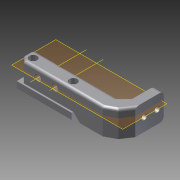
# Autodesk Inventor part: Support Extruder
Saved by Autodesk Inventor 2012 (Build 160160000, 160)
## iProperties
Created: 2013-02-25
Part Number: Support Extruder
Material: Default
Document SubType Name: Modeling
Designer: mce
Density: 1 g/cm^3
Author: mce
Autodesk Inventor part; units mm, degrees
ref_plane "YZ Plane" through (0, 0, 0) normal (1, 0, 0) x (0, 1, 0)
ref_plane "XZ Plane" through (0, 0, 0) normal (0, 1, 0) x (-1, 0, 0)
ref_plane "XY Plane" through (0, 0, 0) normal (0, 0, 1) x (1, 0, 0)
sketch "Sketch1" plane through (0, 0, 0) normal (0, 0, 1) x (1, 0, 0)
  line L0 (3.2057, 1.8441) -> (73.2057, 1.8441)
  line L1 (73.2057, 1.8441) -> (81.2057, 13.8441)
  line L2 (3.2057, 13.8441) -> (3.2057, 1.8441)
  line L3 (73.2057, 18.8441) -> (73.2057, 35.8441)
  line L4 (73.2057, 35.8441) -> (81.2057, 35.8441)
  line L5 (81.2057, 35.8441) -> (81.2057, 13.8441)
  arc A0 (18.1952, 13.8441) -> (30.6162, 13.8441) centre (24.4057, 23.0441) ccw
  line L6 (68.2057, 13.8441) -> (30.6162, 13.8441)
  line L7 (18.1952, 13.8441) -> (3.2057, 13.8441)
  line L8 (73.2057, 18.8441) -> (68.2057, 13.8441)
  circle A1 centre (8.9057, 7.3441) radius 1.6
  circle A2 centre (39.9057, 7.3441) radius 1.6
  point P0 (73.2057, 13.8441)
  dimension "d0" = 70
  dimension "d2" = 8
  dimension "d4" = 21.2
  dimension "d5" = 21.2
  dimension "d6" = 22.2
  dimension "d7" = 12
  dimension "d8" = 22
  dimension "d9" = 5
  dimension "d10" = 5
  dimension "d11" = 31
  dimension "d12" = 5.7
  dimension "d13" = 3.2
  dimension "d14" = 5.5
  constraints: 18 end point, 4 point on line, 3 centre point, 2 point on circle, 1 collinear, 1 equal radius, 1 horizontal, 1 horizontal alignment, 1 vertical, 1 other
  measures "d0" distance between parallel lines of L2 L3
  measures "d2" distance between parallel lines of L3 L5
  measures "d4" distance from line of L0 A0.centre
  measures "d5" distance from line of L2 A0.centre
  measures "d6" diameter of A0
  measures "d7" distance between parallel lines of L7 L0
  measures "d8" distance between parallel lines of L4 L6
  measures "d9" distance of L3.start point (73.206, 13.844)
  measures "d10" distance of L6.start point (73.206, 13.844)
  measures "d11" distance of A1.centre A2.centre
  measures "d12" distance from line of L2 A1.centre
  measures "d13" diameter of A1
  measures "d14" distance from line of A1.centre L0
extrude "Extrusion1" add sketch "Sketch1" along normal blind 20
sketch "Sketch2" plane through (81.2057, 13.8441, 0) normal (1, 0, 0) x (0, 0, -1)
  line L0 (-20, 22) -> (-20, 0) projected
  line L1 (0, 22) -> (-20, 22) projected
  circle A0 centre (-10, 17) radius 2.1
  circle A1 centre (-10, 7) radius 2.1
  point P0 (0, -13.8441)
  dimension "d17" = 10
  dimension "d18" = 4.2
  dimension "d19" = 10
  dimension "d20" = 5
  constraints: 2 centre point, 1 equal radius, 1 vertical alignment
  measures "d17" distance from line of L0 A0.centre
  measures "d18" diameter of A0
  measures "d19" distance of A0.centre A1.centre
  measures "d20" distance from line of L1 A0.centre
extrude "Extrusion2" cut sketch "Sketch2" against normal up to next
sketch "Sketch3" plane through (73.2057, 18.8441, 0) normal (-1, 0, 0) x (0, 0, 1)
  circle A0 centre (10, 2) radius 2.1 projected
  circle A1 centre (10, 12) radius 2.1 projected
  arc A2 (13.75, 12) -> (6.25, 12) centre (10, 12) ccw
  arc A3 (6.25, 2) -> (13.75, 2) centre (10, 2) ccw
  line L0 (6.25, 12) -> (6.25, 2)
  line L1 (13.75, 12) -> (13.75, 2)
  point P0 (0, -18.8441)
  dimension "d23" = 7.5
  constraints: 4 end point, 4 point on circle, 3 tangent, 2 centre point, 2 coincident, 1 equal radius, 1 parallel
  measures "d23" diameter of A2
extrude "Extrusion3" cut sketch "Sketch3" along normal blind 10 and the other way blind 4 contours A0 | L1 A3 L0 A2
sketch "Sketch4" plane through (3.2057, 1.8441, 0) normal (0, -1, 0) x (1, 0, 0)
  line L0 (0, 0) -> (0, 20) projected
  line L1 (0, 0) -> (70, 0) projected
  arc A0 (13.7, 8.5) -> (13.7, 3.5) centre (13.7, 6) ccw
  arc A1 (28.7, 3.5) -> (28.7, 8.5) centre (28.7, 6) ccw
  line L2 (13.7, 8.5) -> (28.7, 8.5)
  line L3 (13.7, 3.5) -> (28.7, 3.5)
  point P0 (-3.2057, 0)
  dimension "d28" = 5
  dimension "d29" = 6
  dimension "d30" = 15
  dimension "d31" = 13.7
  constraints: 4 end point, 4 point on circle, 2 centre point, 2 horizontal, 1 equal radius, 1 horizontal alignment
  measures "d28" diameter of A0
  measures "d29" distance from line of L1 A0.centre
  measures "d30" distance of A1.centre A0.centre
  measures "d31" distance from line of L0 A0.centre
extrude "Extrusion4" [suppressed]
sketch "Sketch5" plane through (3.2057, 1.8441, 0) normal (0, -1, 0) x (1, 0, 0)
  line L0 (0, 0) -> (0, 20) projected
  line L1 (0, 0) -> (70, 0) projected
  circle A0 centre (14.7, 14) radius 1
  circle A1 centre (27.7, 14) radius 1
  point P0 (-3.2057, 0)
  dimension "d34" = 13
  dimension "d35" = 14.7
  dimension "d36" = 14
  dimension "d37" = 2
  constraints: 2 centre point, 1 equal radius, 1 horizontal alignment
  measures "d34" distance of A1.centre A0.centre
  measures "d35" distance from line of L0 A0.centre
  measures "d36" distance from line of L1 A0.centre
  measures "d37" diameter of A0
extrude "Extrusion5" cut sketch "Sketch5" against normal up to next
sketch "Sketch6" plane through (3.2057, 1.8441, 0) normal (0, -1, 0) x (1, 0, 0)
  circle A0 centre (27.7, 14) radius 1 projected
  circle A1 centre (14.7, 14) radius 1 projected
  circle A2 centre (14.7, 14) radius 2.1
  circle A3 centre (27.7, 14) radius 2.1
  point P0 (-3.2057, 0)
  dimension "d40" = 4.2
  constraints: 2 centre point, 2 coincident, 1 equal radius
  measures "d40" diameter of A2
extrude "Extrusion6" cut sketch "Sketch6" against normal blind 4
chamfer "Chamfer1" distance 3 angle 30 2 edges at (31.5017, 13.8441, 13.197) (31.5017, 13.8441, 14.803) measured on face at (31.5017, 13.3441, 14.803) measured on face at (31.5017, 13.3441, 13.197)
chamfer "Chamfer2" distance 3 angle 30 1 edges at (16.9057, 13.8441, 14) measured on face at (16.9057, 13.3441, 14)
chamfer "Chamfer3" distance 5 angle 45 1 edges at (73.2057, 1.8441, 10)
chamfer "Chamfer4" distance 4 angle 45 1 edges at (3.2057, 1.8441, 10)
fillet "Fillet1" radius 3 2 edges at (77.2057, 35.8441, 20) (77.2057, 35.8441, 0)
fillet "Fillet2" radius 3 1 edges at (49.4109, 13.8441, 20)
ref_plane "Work Plane1" through (0, 0, 14) normal (0, 0, 1) x (1, 0, 0)
sketch "Sketch10" plane through (0, 0, 14) normal (0, 0, 1) x (1, 0, 0)
  line L0 (15.8057, 1.8441) -> (15.8057, 1.0941)
  line L1 (15.8057, 1.0941) -> (15.1562, 1.4691)
  line L2 (15.1562, 1.4691) -> (15.8057, 1.8441)
  line L3 (13.7777, 1.4691) -> (17.3129, 1.4691) construction
  line L4 (20.0057, 1.8441) -> (15.8057, 1.8441) projected
  point P0 (0, 0)
  dimension "d80" = 60
  dimension "d81" = 0.75
  dimension "d82" = 0
  constraints: 8 end point, 2 point on line, 1 horizontal, 1 symmetric about line
  measures "d80" angle of L1 L2
  measures "d81" distance of L0.start L0.end
  measures "d82" distance of L0.start L4.end
coil "Coil2" sketch "Sketch10" operation cut axis through (17.9057, 1.8441, 14) along (0, 1, 0) pitch 0.8 turns 5.25 hand right
sketch "Sketch12" plane through (0, 0, 14) normal (0, 0, 1) x (1, 0, 0)
  line L0 (28.8057, 1.8441) -> (28.1562, 1.4691)
  line L1 (28.1562, 1.4691) -> (28.8057, 1.0941)
  line L2 (28.8057, 1.0941) -> (28.8057, 1.8441)
  line L3 (26.005, 1.4691) -> (30.2865, 1.4691) construction
  line L4 (33.0057, 1.8441) -> (28.8057, 1.8441) construction
  point P0 (0, 0)
  dimension "d94" = 60
  dimension "d95" = 0.75
  dimension "d96" = 0
  constraints: 8 end point, 2 point on line, 1 horizontal, 1 symmetric about line
  measures "d94" angle of L0 L1
  measures "d95" distance of L1.end L0.start
  measures "d96" distance of L0.start L4.end
coil "Coil3" sketch "Sketch12" operation cut axis through (30.9057, 1.8441, 14) along (0, 1, 0) pitch 0.8 turns 5.25 hand right
sketch "Sketch13" plane through (0, 0, 20) normal (0, 0, 1) x (1, 0, 0)
  circle A0 centre (39.9057, 7.3441) radius 1.6 projected
  circle A1 centre (8.9057, 7.3441) radius 1.6 projected
  circle A2 centre (8.9057, 7.3441) radius 3
  circle A3 centre (39.9057, 7.3441) radius 3
  point P0 (0, 0)
  dimension "d105" = 6
  constraints: 2 centre point, 2 coincident, 1 equal radius
  measures "d105" diameter of A2
extrude "Extrusion9" cut sketch "Sketch13" against normal blind 4
fillet "Fillet3" radius 2 7 edges at (69.2057, 14.8441, 20) (73.2057, 34.9654, 19.1213) (73.2057, 35.8441, 10) (73.2057, 34.9654, 0.8787) (73.2057, 25.8441, 0) (73.2057, 25.8441, 20) (70.7057, 16.3441, 0)
fillet "Fillet4" radius 2 7 edges at (37.7057, 1.8441, 20) (72.0924, 3.9242, 20) (78.5924, 9.9242, 20) (5.2057, 3.8441, 20) (3.2057, 12.9654, 19.1213) (3.2057, 8.3441, 20) (3.2057, 13.8441, 8.5)
sketch "Sketch14" plane through (0, 0, 0) normal (0, 0, -1) x (-1, 0, 0)
  circle A0 centre (-8.9057, 7.3441) radius 1.6 projected
  circle A1 centre (-39.9057, 7.3441) radius 1.6 projected
  line L0 (-71.0341, 13.8441) -> (-30.6162, 13.8441) projected
  line L1 (-7.2057, 1.8441) -> (-68.2057, 1.8441) projected
  line L2 (-3.2057, 11.8441) -> (-3.2057, 5.8441) projected
  line L3 (-45.6057, 18.8441) -> (1.7943, 18.8441)
  line L4 (1.7943, 18.8441) -> (1.7943, -3.1559)
  line L5 (1.7943, -3.1559) -> (-45.6057, -3.1559)
  line L6 (-45.6057, -3.1559) -> (-45.6057, 18.8441)
  point P0 (0, 0)
  dimension "d110" = 5
  dimension "d111" = 5
  dimension "d112" = 5
  dimension "d113" = 42.4
  constraints: 8 end point
  measures "d110" distance between parallel lines of L3 L0
  measures "d111" distance between parallel lines of L5 L1
  measures "d112" distance between parallel lines of L4 L2
  measures "d113" distance between parallel lines of L6 L2
extrude "Extrusion10" cut sketch "Sketch14" against normal blind 5
chamfer "Chamfer5" distance 5 angle 45 1 edges at (45.6057, 7.8441, 0)
sketch "Sketch16" plane through (30.9057, 13.8441, 14) normal (0, 1, 0) x (1, 0, 0)
  line L0 (14.7, 9) -> (-0.2895, 9) projected
  line L1 (40.1284, 14) -> (19.7, 14) projected
  line L2 (-28.2, 14) -> (14.2, 14)
  line L3 (14.2, 14) -> (14.2, 9.25)
  line L4 (14.2, 9.25) -> (-28.2, 9.25)
  line L5 (-28.2, 9.25) -> (-28.2, 14)
  line L6 (-27.7, 9) -> (-27.7, -3) projected
  point P0 (-30.9057, 14)
  dimension "d119" = 0.5
  dimension "d121" = 0.25
  dimension "d122" = 0.5
  constraints: 8 end point, 1 collinear
  measures "d119" distance from line of L3 L0.start
  measures "d121" distance between parallel lines of L4 L0
  measures "d122" distance between parallel lines of L5 L6
extrude "Extrusion11" add sketch "Sketch16" against normal blind 13 and the other way blind 1
sketch "Sketch17" plane through (45.1057, 0.8441, 0) normal (0, 0, -1) x (-1, 0, 0)
  line L0 (0, 0) -> (42.4, 0) projected
  line L1 (42.4, 0) -> (42.4, 14) projected
  line L2 (42.4, 14) -> (0, 14) projected
  line L3 (0, 14) -> (0, 0) projected
  line L4 (1.5, 12.5) -> (40.9, 12.5)
  line L5 (40.9, 12.5) -> (40.9, 1.5)
  line L6 (40.9, 1.5) -> (1.5, 1.5)
  line L7 (1.5, 1.5) -> (1.5, 12.5)
  point P0 (45.1057, -0.8441)
  dimension "d127" = 1.5
  dimension "d128" = 1.5
  dimension "d129" = 1.5
  dimension "d130" = 1.5
  constraints: 8 end point
  measures "d127" distance between parallel lines of L2 L4
  measures "d128" distance between parallel lines of L0 L6
  measures "d129" distance between parallel lines of L3 L7
  measures "d130" distance between parallel lines of L1 L5
extrude "Extrusion12" cut sketch "Sketch17" against normal blind 3.5 contours L4 L5 L6 L7
equation "\"d10\" = d9"
equation "\"d128\" = d127"
equation "\"d129\" = d127"
equation "\"d130\" = d127"
body "Solid1"
